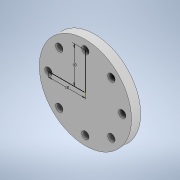
# Autodesk Inventor part: Slit_disk
Saved by Autodesk Inventor 2020 (Build 240168000, 168)
## iProperties
Created: 2021-05-05
Part Number: Slit_disk
Material: 一般
Document SubType Name: Modeling
Designer: owner
Density: 1 g/cm^3
Appearance: 既定
Author: owner
Autodesk Inventor part; units mm, degrees
ref_plane "YZ Plane" through (0, 0, 0) normal (1, 0, 0) x (0, 1, 0)
ref_plane "XZ Plane" through (0, 0, 0) normal (0, 1, 0) x (-1, 0, 0)
ref_plane "XY Plane" through (0, 0, 0) normal (0, 0, 1) x (1, 0, 0)
sketch "スケッチ1" plane through (0, 0, 0) normal (0, 0, 1) x (1, 0, 0)
  circle A0 centre (0, 0) radius 12.5
  dimension "d0" = 25
  constraints: 1 centre point, 1 coincident
  measures "d0" diameter of A0
extrude "押し出し1" add sketch "スケッチ1" along normal blind 2.5
sketch "スケッチ2" plane through (0, 0, 2.5) normal (0, 0, 1) x (1, 0, 0)
  line L0 (0, 0) -> (0, 10)
  dimension "d3" = 10
  constraints: 2 end point, 1 vertical
  measures "d3" distance of L0.start L0.end
sketch "スケッチ3" plane through (0, 0, 2.5) normal (0, 0, 1) x (1, 0, 0)
  circle A0 centre (0, 9.9998) radius 1
  line L0 (0, 0) -> (0, -10)
  dimension "d4" = 2
  dimension "d5" = 10
  constraints: 2 end point, 1 centre point, 1 vertical
  measures "d4" diameter of A0
  measures "d5" distance of L0.start L0.end
sketch "スケッチ4" plane through (0, 0, 2.5) normal (0, 0, 1) x (1, 0, 0)
  circle A0 centre (0, -10) radius 1
  point P0 (0, 0)
  dimension "d6" = 2
  constraints: 1 centre point
  measures "d6" diameter of A0
sketch "スケッチ5" plane through (0, 0, 2.5) normal (0, 0, 1) x (1, 0, 0)
  line L0 (0, 0) -> (-10, 0)
  dimension "d7" = 10
  constraints: 2 end point, 1 horizontal
  measures "d7" distance of L0.start L0.end
sketch "スケッチ6" plane through (0, 0, 2.5) normal (0, 0, 1) x (1, 0, 0)
  circle A0 centre (-10.0003, 0) radius 1
  line L0 (0, 0) -> (10, 0)
  circle A1 centre (10, 0) radius 1
  dimension "d8" = 2
  dimension "d9" = 10
  dimension "d10" = 2
  constraints: 2 centre point, 2 end point, 1 coincident, 1 horizontal
  measures "d8" diameter of A0
  measures "d9" distance of L0.start L0.end
  measures "d10" diameter of A1
extrude "押し出し2" cut sketch "スケッチ3" against normal blind 2.5
extrude "押し出し3" cut sketch "スケッチ6" against normal blind 2.5
extrude "押し出し4" cut sketch "スケッチ4" against normal blind 2.5
sketch "スケッチ7" plane through (0, 0, 2.5) normal (0, 0, 1) x (1, 0, 0)
  line L0 (0, 0) -> (7.0711, 7.0711)
  line L1 (0, 0) -> (10, 0) construction
  line L2 (0, 0) -> (-7.0711, 7.0711)
  line L3 (0, 0) -> (10, 0) construction
  circle A0 centre (-7.0711, 7.0711) radius 1
  circle A1 centre (7.0711, 7.0711) radius 1
  dimension "d17" = 10
  dimension "d18" = 45
  dimension "d19" = 10
  dimension "d20" = 135
  dimension "d21" = 2
  dimension "d22" = 2
  constraints: 8 end point, 2 centre point, 2 coincident, 2 equal length, 2 horizontal
  measures "d17" distance of L0.start L0.end
  measures "d18" angle of L1 L0
  measures "d19" distance of L0.start L2.end
  measures "d20" angle of L3 L2
  measures "d21" diameter of A0
  measures "d22" diameter of A1
sketch "スケッチ8" plane through (0, 0, 2.5) normal (0, 0, 1) x (1, 0, 0)
  line L0 (0, 0) -> (-7.0711, -7.0711)
  line L1 (0, 0) -> (10, 0) construction
  circle A0 centre (-7.0711, -7.0711) radius 1
  line L2 (0, 0) -> (7.0711, -7.0711)
  line L3 (0, 0) -> (10, 0) construction
  circle A1 centre (7.0711, -7.0711) radius 1
  dimension "d23" = 10
  dimension "d24" = 135
  dimension "d25" = 2
  dimension "d26" = 10
  dimension "d27" = 45
  dimension "d28" = 2
  constraints: 8 end point, 2 centre point, 2 coincident, 2 equal length, 2 horizontal
  measures "d23" distance of L0.start L0.end
  measures "d24" angle of L0 L1
  measures "d25" diameter of A0
  measures "d26" distance of L0.start L2.end
  measures "d27" angle of L2 L3
  measures "d28" diameter of A1
extrude "押し出し5" cut sketch "スケッチ7" against normal blind 2.5
extrude "押し出し6" cut sketch "スケッチ8" against normal blind 2.5
sketch "スケッチ9" plane through (0, 0, 2.5) normal (0, 0, 1) x (1, 0, 0)
  point P0 (0, 0)
